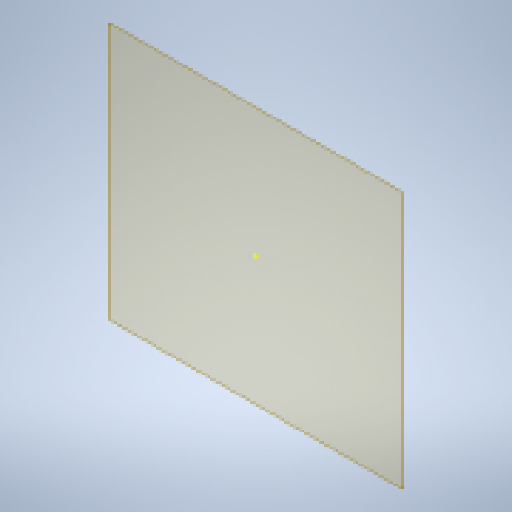
# Autodesk Inventor part: стенка держит стенку
Saved by Autodesk Inventor 2024.2 (Build 282272000, 272)
## iProperties
Created: 2026-02-01
Part Number: стенка держит стенку
Material: Типовые
Document SubType Name: Modeling
Designer: katya_notebook
Density: 1 g/cm^3
Appearance: Прозрачный — зеленый 1
Author: katya_notebook
Autodesk Inventor part; units mm, degrees
ref_plane "YZ Plane" through (0, 0, 0) normal (1, 0, 0) x (0, 1, 0)
ref_plane "XZ Plane" through (0, 0, 0) normal (0, 1, 0) x (-1, 0, 0)
ref_plane "XY Plane" through (0, 0, 0) normal (0, 0, 1) x (1, 0, 0)
ref_plane "РабПлоскость1" through (0, 0, 0) normal (0, 0, 1) x (1, 0, 0)
sketch "Эскиз1" plane through (0, 0, 0) normal (0, 0, 1) x (1, 0, 0)
  line L0 (111.5, 97.5) -> (111.5, -97.5) projected
  line L1 (65.5, 97.5) -> (111.5, 97.5) projected
  line L2 (65.5, 63.1836) -> (65.5, 97.5) projected
  line L3 (65.5, 63.1836) -> (57.5, 63.1836) projected
  line L4 (57.5, 53.1836) -> (57.5, 63.1836) projected
  line L5 (65.5, 53.1836) -> (57.5, 53.1836) projected
  line L6 (65.5, -53.1539) -> (65.5, 53.1836) projected
  line L7 (65.5, -53.1539) -> (57.5, -53.1539) projected
  line L8 (57.5, -63.1539) -> (57.5, -53.1539) projected
  line L9 (65.5, -63.1539) -> (57.5, -63.1539) projected
  line L10 (65.5, -97.5) -> (65.5, -63.1539) projected
  line L11 (111.5, -97.5) -> (65.5, -97.5) projected
  line L12 (65.5, 53.1836) -> (111.5, 53.1836)
  line L13 (111.5, 53.1836) -> (111.5, 47.1836)
  line L14 (111.5, 47.1836) -> (65.5, 47.1836)
  line L15 (65.5, 47.1836) -> (65.5, 53.1836)
  line L16 (65.5, -53.1539) -> (111.5, -53.1539)
  line L17 (111.5, -53.1539) -> (111.5, -47.1539)
  line L18 (111.5, -47.1539) -> (65.5, -47.1539)
  line L19 (65.5, -47.1539) -> (65.5, -53.1539)
  point P0 (0, 0)
  dimension "d0" = 6
  dimension "d1" = 6
  constraints: 16 end point, 4 parallel, 2 horizontal, 2 perpendicular, 2 point on line
  measures "d0" distance of L5.start L14.end
  measures "d1" distance of L18.end L6.start
ref_plane "РабПлоскость2" through (57.5, -97.5, 20) normal (0, 0, -1) x (0, 1, 0)
extrude "Выдавливание1" add sketch "Эскиз1" along normal up to surface (20 mm away) contours L0 L16 L6 L18
sketch "Эскиз2" plane through (65.5, -53.1539, 0) normal (0, -1, 0) x (1, 0, 0)
  line L0 (46, 24) -> (0, 24) projected
  line L1 (0, 20) -> (46, 20) projected
  line L2 (0, 20) -> (12, 20)
  line L3 (12, 20) -> (12, 24)
  line L4 (12, 24) -> (0, 24)
  line L5 (0, 24) -> (0, 20)
  line L6 (46, 20) -> (34, 20)
  line L7 (34, 20) -> (34, 24)
  line L8 (34, 24) -> (46, 24)
  line L9 (46, 24) -> (46, 20)
  point P0 (-65.5, 0)
  point P1 (34, 20)
  dimension "d4" = 12
  dimension "d5" = 12
  constraints: 16 end point, 4 parallel, 2 horizontal, 2 perpendicular, 2 point on line
  measures "d4" distance of L0.end L3.end
  measures "d5" distance of L0.start L7.end
sketch "Эскиз3" plane through (65.5, -53.1539, 0) normal (0, -1, 0) x (1, 0, 0)
  line L0 (31, 10.1574) -> (31, 5.1574)
  line L1 (26.25, 14.0145) -> (19.75, 14.0145)
  line L2 (19.75, 14.0145) -> (19.75, 16.5145)
  line L3 (19.75, 16.5145) -> (26.25, 16.5145)
  line L4 (26.25, 16.5145) -> (26.25, 14.0145)
  line L5 (24.75, 20) -> (21.25, 20)
  line L6 (21.25, 20) -> (21.25, 7.3147)
  line L7 (21.25, 7.3147) -> (24.75, 7.3147)
  line L8 (24.75, 7.3147) -> (24.75, 20)
  line L9 (24.75, 20) -> (21.25, 7.3147) construction
  line L10 (21.25, 20) -> (24.75, 7.3147) construction
  line L11 (24.75, 20) -> (21.25, 16.5145)
  line L12 (24.75, 16.5145) -> (21.25, 20)
  line L13 (46, 20) -> (0, 20) projected
  point P0 (-65.5, 0)
  point P1 (23, 13.6574)
  point P2 (23, 20)
  point P3 (21.25, 14.0145)
  point P4 (24.75, 14.0145)
  dimension "d6" = 6.5
  dimension "d7" = 2.5
  dimension "d10" = 4.75
  dimension "d12" = 3.5
  dimension "d13" = 3.25
  constraints: 26 end point, 4 midpoint, 4 parallel, 4 point on line, 2 horizontal, 2 perpendicular
  measures "d6" distance of L4.end L1.end
  measures "d7" distance of L4.start L4.end
  measures "d10" distance between parallel lines of L0 L4
  measures "d12" distance of L7.start L7.end
  measures "d13" distance from line of L4 point (23, 13.657)
extrude "Выдавливание2" add sketch "Эскиз2" against normal blind 6 contours L9 L1 L7 L0 | L3 L1 L5 L0
extrude "Выдавливание3" cut sketch "Эскиз3" against normal blind 6
sketch "Эскиз4" plane through (65.5, -53.1539, 0) normal (0, -1, 0) x (1, 0, 0)
  line L0 (46, 0) -> (0, 0) projected
  line L1 (12, 0) -> (34, 0)
  line L2 (34, 0) -> (34, -4)
  line L3 (34, -4) -> (12, -4)
  line L4 (12, -4) -> (12, 0)
  point P0 (-65.5, 0)
  point P1 (34, 0)
  dimension "d18" = 12
  dimension "d19" = 12
  dimension "d20" = 4
  constraints: 8 end point, 2 parallel, 1 horizontal, 1 perpendicular, 1 point on line
  measures "d18" distance of L1.start L0.end
  measures "d19" distance of L0.start L1.end
  measures "d20" distance of L3.end L1.start
extrude "Выдавливание4" add sketch "Эскиз4" against normal blind 6
sketch "Эскиз5" plane through (65.5, -53.1539, 24) normal (0, -1, 0) x (1, 0, 0)
  line L0 (9.25, -21.8) -> (2.75, -21.8)
  line L1 (2.75, -21.8) -> (2.75, -19.3)
  line L2 (2.75, -19.3) -> (9.25, -19.3)
  line L3 (9.25, -19.3) -> (9.25, -21.8)
  line L4 (4.25, -12.6005) -> (7.75, -12.6005)
  line L5 (7.75, -12.6005) -> (7.75, -24)
  line L6 (7.75, -24) -> (4.25, -24)
  line L7 (4.25, -24) -> (4.25, -12.6005)
  line L8 (4.25, -12.6005) -> (7.75, -24) construction
  line L9 (7.75, -12.6005) -> (4.25, -24) construction
  line L10 (0, -24) -> (12, -24) projected
  line L11 (43.25, -19.3) -> (43.25, -21.8)
  line L12 (41.75, -24) -> (38.25, -24)
  line L13 (41.75, -12.6) -> (41.75, -24)
  line L14 (43.25, -21.8) -> (36.75, -21.8)
  line L15 (36.75, -19.3) -> (43.25, -19.3)
  line L16 (38.25, -12.6) -> (41.75, -24) construction
  line L17 (38.25, -12.6) -> (41.75, -12.6)
  line L18 (41.75, -12.6) -> (38.25, -24) construction
  line L19 (36.75, -21.8) -> (36.75, -19.3)
  line L20 (38.25, -24) -> (38.25, -12.6)
  line L21 (34, -24) -> (46, -24) projected
  point P0 (-65.5, -24)
  point P1 (6, -18.3002)
  point P2 (6, -24)
  point P3 (40, -18.3)
  point P4 (42.6795, -22.1366)
  point P5 (40, -24)
  point P6 (38.25, -19.3)
  point P7 (38.25, -21.8)
  point P8 (41.75, -21.8)
  point P9 (41.75, -19.3)
  point P10 (4.25, -19.3)
  point P11 (4.25, -21.8)
  point P12 (7.75, -21.8)
  point P13 (7.75, -19.3)
  dimension "d23" = 6.5
  dimension "d24" = 2.5
  dimension "d29" = 3.5
  dimension "d30" = 3.25
  dimension "d31" = 2.2
  dimension "d32" = 6.5
  dimension "d33" = 2.5
  dimension "d34" = 3.5
  dimension "d35" = 3.25
  dimension "d36" = 2.2
  dimension "d39" = 6.7
  constraints: 40 end point, 8 midpoint, 8 parallel, 4 horizontal, 4 perpendicular
  measures "d23" distance of L3.end L0.end
  measures "d24" distance of L3.start L3.end
  measures "d29" distance of L6.start L6.end
  measures "d30" distance from line of L3 point (6, -18.3)
  measures "d31" distance from line of L0 L6.start
  measures "d32" distance of L11.end L14.end
  measures "d33" distance of L11.start L11.end
  measures "d34" distance of L12.start L12.end
  measures "d35" distance from line of L11 point (40, -18.3)
  measures "d36" distance from line of L14 L12.start
  measures "d39" distance from line of L15 L16.start
extrude "Выдавливание5" cut sketch "Эскиз5" against normal blind 6
